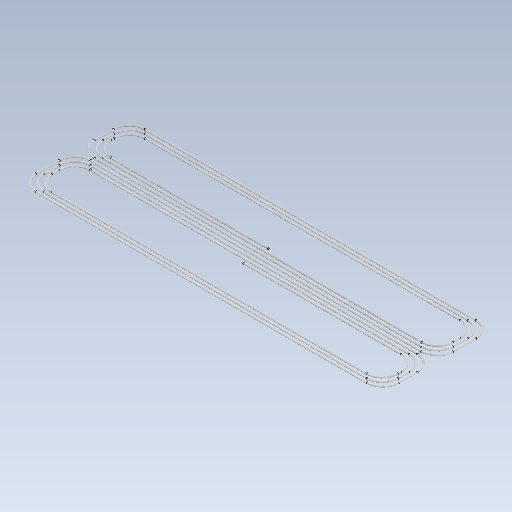
# Autodesk Inventor part: coil
Saved by Autodesk Inventor 2021 (Build 250183000, 183)
## iProperties
Created: 2022-01-18
Part Number: coil
Material: Generic
Document SubType Name: Modeling
Designer: avan411
Density: 1 g/cm^3
Appearance: Default
Author: avan411
Autodesk Inventor part; units mm, degrees
ref_plane "YZ Plane" through (0, 0, 0) normal (1, 0, 0) x (0, 1, 0)
ref_plane "XZ Plane" through (0, 0, 0) normal (0, 1, 0) x (-1, 0, 0)
ref_plane "XY Plane" through (0, 0, 0) normal (0, 0, 1) x (1, 0, 0)
sketch "Sketch1" plane through (0, 0, 0) normal (0, 1, 0) x (-1, 0, 0)
  line L0 (0, 0) -> (-500, 0) construction
  line L1 (-500, 0) -> (-500, -150) construction
  line L2 (-500, -150) -> (500, -150) construction
  line L3 (500, -150) -> (500, -11.4333) construction
  line L4 (500, -11.4333) -> (-488.75, -11.4333) construction
  line L5 (-488.75, -11.4333) -> (-488.75, -139.25) construction
  line L6 (-488.75, -139.25) -> (488.75, -139.25) construction
  line L7 (488.75, -139.25) -> (488.75, -22.8667) construction
  line L8 (488.75, -22.8667) -> (-477.5, -22.8667) construction
  line L9 (-477.5, -22.8667) -> (-477.5, -128.5) construction
  line L10 (-477.5, -128.5) -> (477.5, -128.5) construction
  line L11 (477.5, -128.5) -> (477.5, -34.3) construction
  line L12 (477.5, -34.3) -> (0, -34.3) construction
  line L13 (0, 0) -> (0, -11.4333) construction
  line L14 (0, -11.4333) -> (0, -22.8667) construction
  line L15 (0, -22.8667) -> (0, -34.3) construction
  line L16 (0, -128.5) -> (0, -139.25) construction
  line L17 (0, -139.25) -> (0, -150) construction
  line L18 (500, -34.3) -> (488.75, -34.3) construction
  line L19 (488.75, -34.3) -> (477.5, -34.3) construction
  line L20 (-477.5, -22.8667) -> (-488.75, -22.8667) construction
  line L21 (-488.75, -22.8667) -> (-500, -22.8667) construction
  line L22 (0, 0) -> (500, 0)
  line L23 (500, 0) -> (500, 150) construction
  line L24 (500, 150) -> (-500, 150) construction
  line L25 (-500, 150) -> (-500, 11.4333) construction
  line L26 (-500, 11.4333) -> (488.75, 11.4333) construction
  line L27 (488.75, 11.4333) -> (488.75, 139.25) construction
  line L28 (488.75, 139.25) -> (-488.75, 139.25) construction
  line L29 (-488.75, 139.25) -> (-488.75, 22.8667) construction
  line L30 (-488.75, 22.8667) -> (477.5, 22.8667) construction
  line L31 (477.5, 22.8667) -> (477.5, 128.5) construction
  line L32 (477.5, 128.5) -> (-477.5, 128.5) construction
  line L33 (-477.5, 128.5) -> (-477.5, 34.3) construction
  line L34 (-477.5, 34.3) -> (0, 34.3) construction
  line L35 (0, 0) -> (0, 11.4333) construction
  line L36 (0, 11.4333) -> (0, 22.8667) construction
  line L37 (0, 22.8667) -> (0, 34.3) construction
  line L38 (0, 128.5) -> (0, 139.25) construction
  line L39 (0, 139.25) -> (0, 150) construction
  line L40 (-500, 34.3) -> (-488.75, 34.3) construction
  line L41 (-488.75, 34.3) -> (-477.5, 34.3) construction
  line L42 (477.5, 22.8667) -> (488.75, 22.8667) construction
  line L43 (488.75, 22.8667) -> (500, 22.8667) construction
  arc A0 (477.5, -77.3) -> (434.5, -34.3) centre (434.5, -77.3) ccw
  arc A1 (488.75, -65.8667) -> (445.75, -22.8667) centre (445.75, -65.8667) ccw
  arc A2 (500, -54.4333) -> (457, -11.4333) centre (457, -54.4333) ccw
  arc A3 (434.5, -128.5) -> (477.5, -85.5) centre (434.5, -85.5) ccw
  arc A4 (445.75, -139.25) -> (488.75, -96.25) centre (445.75, -96.25) ccw
  arc A5 (457, -150) -> (500, -107) centre (457, -107) ccw
  arc A6 (-434.5, -22.8667) -> (-477.5, -65.8667) centre (-434.5, -65.8667) ccw
  arc A7 (-477.5, 77.3) -> (-434.5, 34.3) centre (-434.5, 77.3) ccw
  arc A8 (-488.75, 65.8667) -> (-445.75, 22.8667) centre (-445.75, 65.8667) ccw
  arc A9 (-500, 54.4333) -> (-457, 11.4333) centre (-457, 54.4333) ccw
  arc A10 (-500, -107) -> (-457, -150) centre (-457, -107) ccw
  arc A11 (-488.75, -96.25) -> (-445.75, -139.25) centre (-445.75, -96.25) ccw
  arc A12 (-477.5, -85.5) -> (-434.5, -128.5) centre (-434.5, -85.5) ccw
  arc A13 (-457, 150) -> (-500, 107) centre (-457, 107) ccw
  arc A14 (-445.75, 139.25) -> (-488.75, 96.25) centre (-445.75, 96.25) ccw
  arc A15 (434.5, 22.8667) -> (477.5, 65.8667) centre (434.5, 65.8667) ccw
  arc A16 (445.75, 11.4333) -> (488.75, 54.4333) centre (445.75, 54.4333) ccw
  arc A17 (457, 0) -> (500, 43) centre (457, 43) ccw
  arc A18 (477.5, 85.5) -> (434.5, 128.5) centre (434.5, 85.5) ccw
  arc A19 (-445.75, -11.4333) -> (-488.75, -54.4333) centre (-445.75, -54.4333) ccw
  arc A20 (-457, 0) -> (-500, -43) centre (-457, -43) ccw
  arc A21 (-434.5, 128.5) -> (-477.5, 85.5) centre (-434.5, 85.5) ccw
  arc A22 (500, 107) -> (457, 150) centre (457, 107) ccw
  arc A23 (488.75, 96.25) -> (445.75, 139.25) centre (445.75, 96.25) ccw
  line L44 (0, -34.3) -> (434.5, -34.3)
  line L45 (434.5, -128.5) -> (-434.5, -128.5)
  line L46 (-434.5, -22.8667) -> (445.75, -22.8667)
  line L47 (445.75, -139.25) -> (-445.75, -139.25)
  line L48 (457, -150) -> (-457, -150)
  line L49 (-445.75, -11.4333) -> (457, -11.4333)
  line L50 (-457, 0) -> (457, 0)
  line L51 (500, -54.4333) -> (500, -107)
  line L52 (488.75, -65.8667) -> (488.75, -96.25)
  line L53 (477.5, -85.5) -> (477.5, -77.3)
  line L54 (-477.5, -65.8667) -> (-477.5, -85.5)
  line L55 (-488.75, -96.25) -> (-488.75, -54.4333)
  line L56 (-500, -43) -> (-500, -107)
  line L57 (-500, 54.4333) -> (-500, 107)
  line L58 (-488.75, 96.25) -> (-488.75, 65.8667)
  line L59 (500, 43) -> (500, 107)
  line L60 (488.75, 96.25) -> (488.75, 54.4333)
  line L61 (477.5, 85.5) -> (477.5, 65.8667)
  line L62 (445.75, 11.4333) -> (-457, 11.4333)
  line L63 (-445.75, 22.8667) -> (434.5, 22.8667)
  line L64 (434.5, 128.5) -> (-434.5, 128.5)
  line L65 (-445.75, 139.25) -> (445.75, 139.25)
  line L66 (457, 150) -> (-457, 150)
  line L67 (-434.5, 34.3) -> (0, 34.3)
  line L68 (-477.5, 85.5) -> (-477.5, 77.3)
  dimension "d5" = 1000
  dimension "d6" = 150
  dimension "d7" = 500
  dimension "d8" = 34.3
  dimension "d9" = 21.5
  dimension "d11" = 22.5
  dimension "d13" = 150
  dimension "d14" = 500
  dimension "d15" = 34.3
  dimension "d16" = 21.5
  dimension "d17" = 22.5
  dimension "d18" = 0
  dimension "d19" = 43
  constraints: 138 end point, 74 point on line, 53 tangent, 48 point on circle, 32 perpendicular, 24 centre point, 23 equal radius, 21 collinear, 12 equal length, 8 parallel, 6 midpoint, 3 horizontal
  measures "d5" distance of L1.end L2.end
  measures "d6" distance of L0.end L1.end
  measures "d7" distance of L0.start L0.end
  measures "d8" distance between parallel lines of L0 L12
  measures "d9" distance between parallel lines of L2 L10
  measures "d11" distance between parallel lines of L1 L9
  measures "d13" distance of L23.start L23.end
  measures "d14" distance of L0.start L23.start
  measures "d15" distance between parallel lines of L22 L34
  measures "d16" distance between parallel lines of L24 L32
  measures "d17" distance between parallel lines of L23 L31
  measures "d18" distance from line of L13 L0.start
  measures "d19" radius of A12
sketch "Sketch2" plane through (0, 0, 0) normal (1, 0, 0) x (0, 1, 0)
  line L0 (-2.15, -32.15) -> (2.15, -32.15) construction
  line L1 (2.15, -32.15) -> (2.15, -36.45) construction
  line L2 (2.15, -36.45) -> (-2.15, -36.45) construction
  line L3 (-2.15, -36.45) -> (-2.15, -32.15) construction
  line L4 (-2.15, -32.15) -> (2.15, -36.45) construction
  line L5 (2.15, -32.15) -> (-2.15, -36.45) construction
  circle A0 centre (0, -34.3) radius 2.15
  point P0 (0, 0)
  dimension "d20" = 4.3
  constraints: 12 end point, 2 midpoint, 2 parallel, 2 perpendicular, 1 centre point, 1 coincident, 1 horizontal
  measures "d20" distance of L0.end L1.end
sweep "Sweep3" add profiles "Sketch2" path "Sketch1" path curves L44 A0 L53 A3 L45 A12 L54 A6 L46 A1 L52 A4 L47 A11 L55 A19 L49 A2 L51 A5 L48 A10 L56 A20 L50 A17 L59 A22 L66 A13 L57 A9 L62 A16 L60 A23 L65 A14 L58 A8 L63 A15 L61 A18 L64 A21 L68 A7 L67
body "Solid3"
